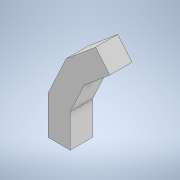
# Autodesk Inventor part: bent_finger_model
Saved by Autodesk Inventor 2021 (Build 250183000, 183)
## iProperties
Created: 2021-03-09
Part Number: bent_finger_model
Material: Generic
Document SubType Name: Modeling
Designer: Charlie
Density: 1 g/cm^3
Appearance: Default
Author: Charlie
Autodesk Inventor part; units mm, degrees
ref_plane "YZ Plane" through (0, 0, 0) normal (1, 0, 0) x (0, 1, 0)
ref_plane "XZ Plane" through (0, 0, 0) normal (0, 1, 0) x (-1, 0, 0)
ref_plane "XY Plane" through (0, 0, 0) normal (0, 0, 1) x (1, 0, 0)
sketch "Sketch1" plane through (0, 0, 0) normal (0, 0, 1) x (1, 0, 0)
  line L0 (-10, -15) -> (10, -15)
  line L1 (10, -15) -> (10, 15)
  line L2 (10, 15) -> (-10, 15) construction
  line L3 (-10, 19.4339) -> (-10, -15)
  line L4 (-10, -15) -> (10, 15) construction
  line L5 (10, -15) -> (-10, 15) construction
  line L6 (10, 15) -> (22.6785, 42.1892)
  line L7 (22.6785, 42.1892) -> (4.5524, 50.6416) construction
  line L8 (6.4262, 54.6601) -> (-10, 19.4339)
  line L9 (9.8228, 57.5101) -> (22.6785, 42.1892) construction
  line L10 (22.6785, 42.1892) -> (45.6599, 61.4729)
  line L11 (45.6599, 61.4729) -> (32.8041, 76.7938)
  line L12 (32.8041, 76.7938) -> (6.4262, 54.6601)
  line L13 (12.6785, 27.1892) -> (32.6785, 57.1892) construction
  line L14 (32.6785, 27.1892) -> (12.6785, 57.1892) construction
  point P0 (0, 0)
  dimension "d3" = 30
  dimension "d4" = 20
  dimension "d5" = 30
  dimension "d6" = 34.4339
  dimension "d9" = 90
  dimension "d10" = 20
  dimension "d12" = 155
  dimension "d13" = 35.2262
  dimension "d14" = 22.1337
  dimension "d15" = 26.3779
  dimension "d16" = 20
  constraints: 30 end point, 5 parallel, 4 midpoint, 3 point on line, 2 perpendicular, 1 horizontal
  measures "d3" distance of L6.start L6.end
  measures "d4" distance of L0.start L0.end
  measures "d5" distance of L0.end L1.end
  measures "d6" distance of L3.start L0.start
  measures "d9" angle of L7 L6
  measures "d10" distance of L11.end L10.end
  measures "d12" angle of L10 L6
  measures "d13" vertical distance of L8.start L3.start
  measures "d14" vertical distance of L11.end L8.start
  measures "d15" horizontal distance of L11.end L8.start
  measures "d16" distance between parallel lines of L6 L8
extrude "Extrusion1" add sketch "Sketch1" along normal blind 20
body "Solid1"
